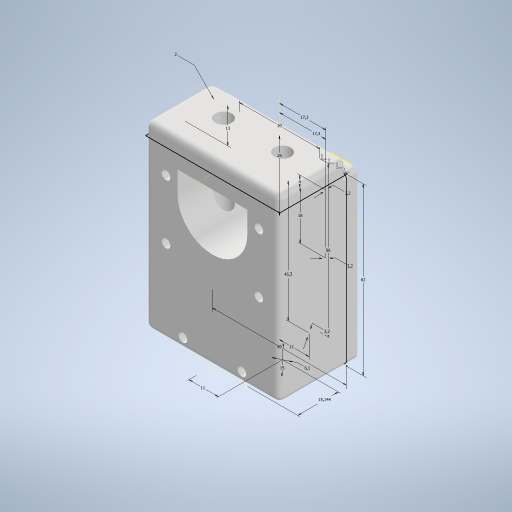
# Autodesk Inventor part: uMule-uchwyt_dx_góra
Saved by Autodesk Inventor 2024.2 (Build 282272000, 272)
## iProperties
Created: 2024-10-21
Part Number: uMule-uchwyt_dx_góra
Material: Ogólny
Document SubType Name: Modeling
Designer: owozn
Density: 1 g/cm^3
Appearance: Domyślna
Author: owozn
Autodesk Inventor part; units mm, degrees
ref_plane "YZ Plane" through (0, 0, 0) normal (1, 0, 0) x (0, 1, 0)
ref_plane "XZ Plane" through (0, 0, 0) normal (0, 1, 0) x (-1, 0, 0)
ref_plane "XY Plane" through (0, 0, 0) normal (0, 0, 1) x (1, 0, 0)
sketch "Szkic1" plane through (0, 0, 0) normal (0, 0, 1) x (1, 0, 0)
  line L0 (-35.5799, 0) -> (35.5799, 0) construction
  line L1 (0, -61.9799) -> (0, 25.9799) construction
  line L2 (-23, 13) -> (23, 13)
  line L3 (25, 11) -> (25, -47)
  line L4 (23, -49) -> (-23, -49)
  line L5 (-25, -47) -> (-25, 11)
  circle A0 centre (17.3, 4) radius 1.6
  circle A1 centre (17.3, -18) radius 1.6
  circle A2 centre (11, -45.3) radius 1.6
  circle A3 centre (-17.3, 4) radius 1.6
  circle A4 centre (-17.3, -18) radius 1.6
  circle A5 centre (-11, -45.3) radius 1.6
  circle A6 centre (0, 0) radius 13
  arc A7 (-23, 13) -> (-25, 11) centre (-23, 11) ccw
  arc A8 (-25, -47) -> (-23, -49) centre (-23, -47) ccw
  arc A9 (23, -49) -> (25, -47) centre (23, -47) ccw
  arc A10 (25, 11) -> (23, 13) centre (23, 11) ccw
  line L6 (-15, -43) -> (15, -43)
  line L7 (15, -43) -> (15, 13)
  line L8 (15, 13) -> (-15, 13)
  line L9 (-15, 13) -> (-15, -43)
  line L10 (-15, -43) -> (15, 13) construction
  line L11 (15, -43) -> (-15, 13) construction
  line L12 (13, 0) -> (13, 13)
  line L13 (-13, 0) -> (-13, 13)
  point P0 (25, -49)
  point P1 (25, 13)
  point P2 (-25, -49)
  point P3 (0, -15)
  point P4 (0, 13)
  dimension "d12" = 26
  dimension "d0" = 50
  dimension "d1" = 62
  dimension "d2" = 13
  dimension "d3" = 3.2
  dimension "d4" = 3.2
  dimension "d5" = 3.2
  dimension "d6" = 17.3
  dimension "d7" = 17.3
  dimension "d8" = 4
  dimension "d9" = 18
  dimension "d10" = 45.3
  dimension "d11" = 11
  dimension "d13" = 2
  dimension "d14" = 30
  dimension "d15" = 56
  constraints: 24 end point, 10 centre point, 10 point on line, 8 point on circle, 8 tangent, 5 symmetric about line, 4 parallel, 3 equal radius, 3 perpendicular, 2 horizontal, 2 midpoint, 1 coincident, 7 other
  measures "d0" distance of point (25, -49) point (-25, -49)
  measures "d1" distance of point (25, 13) point (25, -49)
  measures "d2" distance between parallel lines of L2 L0
  measures "d3" diameter of A0
  measures "d4" diameter of A1
  measures "d5" diameter of A2
  measures "d6" distance from line of A0.centre L1
  measures "d7" distance from line of L1 A1.centre
  measures "d8" distance from line of L0 A0.centre
  measures "d9" distance from line of A1.centre L0
  measures "d10" distance from line of A2.centre L0
  measures "d11" distance from line of L1 A2.centre
  measures "d13" radius of A7
  measures "d14" distance of L8.end L7.end
  measures "d15" distance of L7.end L6.end
extrude "Wyciągnięcie proste1" add sketch "Szkic1" against normal blind 4 contours L2 L9 L6 L7 A10 L3 A9 L4 A8 L5 A7
extrude "Wyciągnięcie proste2" add sketch "Szkic1" along normal blind 25 contours L2 L9 L6 L7 A10 L3 A9 L4 A8 L5 A7 | L2 L13 A6 L12 L7 L6 L9
sketch "Szkic2" plane through (-23, -49, -4) normal (0, -1, 0) x (1, 0, 0)
  line L0 (-12, 4) -> (58, 4) construction
  line L1 (23, -5.8) -> (23, 34.8) construction
  line L2 (10, 29) -> (36, 29) construction
  circle A0 centre (34, 13.856) radius 3.05
  circle A1 centre (34, 13.856) radius 7.5
  circle A2 centre (12, 13.856) radius 3.05
  circle A3 centre (12, 13.856) radius 7.5
  point P0 (23, 4)
  dimension "d21" = 6.1
  dimension "d22" = 15
  dimension "d23" = 11
  dimension "d24" = 15.144
  constraints: 4 centre point, 2 coincident, 2 symmetric about line, 2 other
  measures "d21" diameter of A0
  measures "d22" diameter of A1
  measures "d23" distance from line of L1 A0.centre
  measures "d24" distance from line of L2 A0.centre
extrude "Wyciągnięcie proste4" add sketch "Szkic2" against normal blind 32
sketch "Szkic3" plane through (15, 13, -4) normal (0, 1, 0) x (1, 0, 0)
  line L0 (-15, 5.8) -> (-15, -34.8) construction
  line L1 (-50, -4) -> (20, -4) construction
  line L2 (-40, -4) -> (10, -4)
  line L3 (10, -4) -> (10, -29)
  line L4 (10, -29) -> (-40, -29)
  line L5 (-40, -29) -> (-40, -4)
  line L6 (-40, -4) -> (10, -29) construction
  line L7 (10, -4) -> (-40, -29) construction
  line L8 (0, 0) -> (8, 0) projected
  circle A0 centre (-26, -13.856) radius 3.05 projected
  circle A1 centre (-26, -13.856) radius 7.5
  circle A2 centre (-4, -13.856) radius 7.5
  point P0 (-15, -4)
  point P1 (-15, -16.5)
  dimension "d31" = 50
  dimension "d32" = 25
  dimension "d37" = 15
  constraints: 13 end point, 2 centre point, 2 midpoint, 2 parallel, 2 point on line, 1 coincident, 1 horizontal, 1 perpendicular, 1 symmetric about line, 1 other
  measures "d31" distance of L3.end L4.end
  measures "d32" distance of L2.end L3.end
  measures "d37" diameter of A1
extrude "Wyciągnięcie proste6" add sketch "Szkic3" along normal mid plane 10 contours L2 L3 L4 L5 | A0 | A1 | A2
extrude "Wyciągnięcie proste7" cut sketch "Szkic2" against normal through all contours A0 | A2
fillet "Zaokrąglenie1" radius 2 11 edges at (-25, 14.5, 0) (-25, 18, 12.5) (0, 18, 0) (25, 18, 12.5) (25, 14.5, 0) (0, 18, 25) (24.4142, -48.4142, 25) (0, -49, 25) (-24.4142, -48.4142, 25) (-25, -14.5, 25) (25, -14.5, 25)
